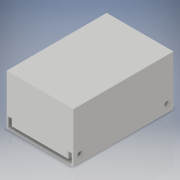
# Autodesk Inventor part: Case
Saved by Autodesk Inventor 2019 (Build 230136000, 136)
## iProperties
Created: 2019-12-10
Part Number: Case
Material: 常规
Document SubType Name: Modeling
Designer: cxcyh
Density: 1 g/cm^3
Appearance: 默认
Author: cxcyh
Autodesk Inventor part; units mm, degrees
ref_plane "YZ Plane" through (0, 0, 0) normal (1, 0, 0) x (0, 1, 0)
ref_plane "XZ Plane" through (0, 0, 0) normal (0, 1, 0) x (-1, 0, 0)
ref_plane "XY Plane" through (0, 0, 0) normal (0, 0, 1) x (1, 0, 0)
sketch "草图2" plane through (0, 0, 0) normal (0, 1, 0) x (-1, 0, 0)
  line L0 (-20, 30) -> (20, 30)
  line L1 (20, 30) -> (20, -30)
  line L2 (20, -30) -> (-20, -30)
  line L3 (-20, -30) -> (-20, 30)
  line L4 (-20, 30) -> (20, -30) construction
  line L5 (20, 30) -> (-20, -30) construction
  point P0 (0, 0)
  dimension "d15" = 40
  dimension "d16" = 60
  constraints: 12 end point, 2 midpoint, 2 parallel, 1 horizontal, 1 perpendicular
  measures "d15" distance of L1.end L2.end
  measures "d16" distance of L0.end L1.end
extrude "拉伸2" add sketch "草图2" along normal blind 30
shell "抽壳1" thickness 2 removed faces 1 at (-6.6667, 0, -10)
sketch "草图3" plane through (-20, 0, 30) normal (0, 0, 1) x (1, 0, 0)
  line L0 (40, 0) -> (0, 0) construction
  line L1 (40, 0) -> (40, 30) construction
  line L2 (0, 30) -> (40, 30) construction
  line L3 (0, 0) -> (0, 30) construction
  line L4 (0, 0) -> (0, 30) construction
  line L5 (40, 0) -> (40, 30) construction
  line L6 (40, 0) -> (0, 0) construction
  line L7 (3, 6.7398) -> (1, 6.7398)
  line L8 (1, 6.7398) -> (1, 0.7398)
  line L9 (0, 1.7398) -> (40, 1.7398) construction
  line L10 (3, 6.7398) -> (3, 2.7398)
  line L11 (40, 30) -> (0, 30) construction
  line L12 (20, 30) -> (20, 0) construction
  line L13 (38, 0) -> (2, 0) projected
  line L14 (3, 2.7398) -> (20, 2.7398)
  line L15 (1, 0.7398) -> (20, 0.7398)
  line L16 (37, 6.7398) -> (39, 6.7398)
  line L17 (39, 6.7398) -> (39, 0.7398)
  line L18 (37, 6.7398) -> (37, 2.7398)
  line L19 (37, 2.7398) -> (20, 2.7398)
  line L20 (39, 0.7398) -> (20, 0.7398)
  point P0 (20, 0)
  dimension "d29" = 2
  dimension "d44" = 5
  dimension "d45" = 2
  dimension "d46" = 6
  dimension "d47" = 40
  constraints: 24 end point, 5 point on line, 4 symmetric about line, 3 horizontal, 3 perpendicular, 2 midpoint
  measures "d29" distance from line of L7.start L8
  measures "d44" distance between parallel lines of L9 L7
  measures "d45" distance between parallel lines of L15 L14
  measures "d46" distance between parallel lines of L15 L7
  measures "d47" diameter of L1 L12
extrude "拉伸3" cut sketch "草图3" against normal blind 58
sketch "草图5" plane through (20, 0, 30) normal (1, 0, 0) x (0, 0, -1)
  line L0 (0, 6.7398) -> (58, 6.7398) construction
  line L1 (0, 0.7398) -> (58, 0.7398) construction
  line L2 (0, 6.7398) -> (2, 6.7398) construction
  line L3 (0, 2.7398) -> (2, 2.7398) construction
  line L4 (0, 2.7398) -> (58, 2.7398) construction
  line L5 (58, 6.7398) -> (2, 6.7398) construction
  line L6 (58, 6.7398) -> (58, 0.7398) construction
  line L7 (0, 0) -> (0, 30) construction
  line L8 (0, 4.7398) -> (58, 4.7398) construction
  circle A0 centre (4, 4.7398) radius 1.5
  line L9 (2, 0.7398) -> (2, 6.7398) construction
  circle A1 centre (56, 4.7398) radius 1.5
  point P0 (30, 0)
  dimension "d48" = 4
  dimension "d49" = 3
  dimension "d51" = 2
  dimension "d52" = 2
  dimension "d53" = 3
  dimension "d54" = 2
  constraints: 8 end point, 6 point on line, 3 perpendicular, 2 centre point, 1 horizontal
  measures "d48" diameter of L0 L8
  measures "d49" diameter of A0
  measures "d51" distance between parallel lines of L7 L9
  measures "d52" distance from line of A0.centre L9
  measures "d53" diameter of A1
  measures "d54" distance of L8.end A1.centre
extrude "拉伸4" cut sketch "草图5" against normal blind 2
mirror "镜像1" about plane through (0, 0, 0) normal (1, 0, 0) of "拉伸4"
sketch "草图7" plane through (-18, 28, 28) normal (0, -1, 0) x (1, 0, 0)
  line L0 (0, 0) -> (36, 0) construction
  line L1 (0, -56) -> (0, 0) construction
  line L2 (36, -56) -> (0, -56) construction
  line L3 (36, 0) -> (36, -56) construction
  line L4 (0.5, -55.5) -> (18.5, -55.5) construction
  line L5 (18.5, -55.5) -> (18.5, -10.5) construction
  line L6 (18.5, -10.5) -> (0.5, -10.5) construction
  line L7 (0.5, -10.5) -> (0.5, -55.5) construction
  circle A0 centre (1.5, -54.5) radius 0.9
  line L8 (3, -56) -> (0, -56)
  line L9 (0, -56) -> (0, -53)
  line L10 (0, -53) -> (3, -53)
  line L11 (3, -53) -> (3, -56)
  line L12 (3, -56) -> (0, -53) construction
  line L13 (0, -56) -> (3, -53) construction
  line L14 (0.5, -55.5) -> (18.5, -10.5) construction
  line L15 (0.5, -10.5) -> (18.5, -55.5) construction
  line L16 (3, -13) -> (0, -13)
  line L17 (0, -13) -> (0, -10)
  line L18 (0, -10) -> (3, -10)
  line L19 (3, -10) -> (3, -13)
  circle A1 centre (1.5, -11.5) radius 0.9
  line L20 (19, -56) -> (16, -56)
  line L21 (16, -56) -> (16, -53)
  line L22 (16, -53) -> (19, -53)
  line L23 (19, -53) -> (19, -56)
  circle A2 centre (17.5, -54.5) radius 0.9
  line L24 (19, -13) -> (16, -13)
  line L25 (16, -13) -> (16, -10)
  line L26 (16, -10) -> (19, -10)
  line L27 (19, -10) -> (19, -13)
  circle A3 centre (17.5, -11.5) radius 0.9
  point P0 (9.5, -33)
  dimension "d70" = 18
  dimension "d71" = 45
  dimension "d79" = 1.8
  dimension "d80" = 1
  dimension "d81" = 1
  dimension "d82" = 3
  dimension "d83" = 3
  dimension "d91" = 43
  dimension "d94" = 16
  dimension "d97" = 1
  dimension "d98" = 1
  constraints: 48 end point, 4 centre point, 4 parallel, 3 horizontal, 3 midpoint, 2 perpendicular, 1 vertical, 30 other
  measures "d70" distance of L6.end L5.end
  measures "d71" distance of L5.end L4.end
  measures "d79" diameter of A0
  measures "d80" distance from line of L7 A0.centre
  measures "d81" distance from line of L4 A0.centre
  measures "d82" distance of L9.end L10.end
  measures "d83" distance of L8.end L9.end
  measures "d91" distance of L8.start L16.start
  measures "d94" distance of L8.start L20.start
  measures "d97" distance from line of L5 A2.centre
  measures "d98" distance from line of L6 A3.centre
sketch "草图9" plane through (20, 0, -30) normal (0, 0, -1) x (-1, 0, 0)
  line L0 (37.5, 28) -> (19.5, 28) construction
  line L1 (32, 24.8) -> (25, 24.8)
  line L2 (25, 24.8) -> (25, 28)
  line L3 (25, 28) -> (32, 28)
  line L4 (32, 28) -> (32, 24.8)
  line L5 (32, 24.8) -> (25, 28) construction
  line L6 (25, 24.8) -> (32, 28) construction
  point P0 (20, 0)
  point P1 (28.5, 26.4)
  dimension "d99" = 18
  dimension "d100" = 7
  dimension "d101" = 3.2
  dimension "d102" = 1.6
  dimension "d103" = 9
  constraints: 12 end point, 2 midpoint, 2 parallel, 1 horizontal, 1 perpendicular
  measures "d99" distance of L0.start L0.end
  measures "d100" distance of L2.end L3.end
  measures "d101" distance of L1.end L2.end
  measures "d102" distance from line of L0 point (28.5, 26.4)
  measures "d103" horizontal distance of L0.end point (28.5, 26.4)
extrude "拉伸5" add sketch "草图7" along normal blind 3.2
extrude "拉伸6" cut sketch "草图9" against normal blind 2
sketch "草图10" plane through (20, 0, -30) normal (0, 0, -1) x (-1, 0, 0)
  line L0 (32, 28) -> (32, 24.8) construction
  line L1 (32, 24.8) -> (25, 24.8) construction
  line L2 (25, 24.8) -> (25, 28) construction
  line L3 (25, 28) -> (32, 28) construction
  line L4 (40, 0) -> (0, 0) construction
  line L5 (40, 0) -> (40, 30) construction
  line L6 (0, 30) -> (40, 30) construction
  line L7 (0, 0) -> (0, 30) construction
  line L8 (25, 28) -> (25, 24.8) construction
  line L9 (25, 24.8) -> (32, 24.8) construction
  line L10 (32, 24.8) -> (32, 28) construction
  line L11 (32, 28) -> (35, 28) construction
  line L12 (35, 28) -> (35, 24.8) construction
  line L13 (35, 24.8) -> (38, 24.8) construction
  line L14 (38, 6.7398) -> (38, 24.8) construction
  line L15 (39, 6.7398) -> (38, 6.7398) construction
  line L16 (39, 0.7398) -> (39, 6.7398) construction
  line L17 (38, 0.7398) -> (39, 0.7398) construction
  line L18 (38, 0) -> (38, 0.7398) construction
  line L19 (2, 0) -> (38, 0) construction
  line L20 (2, 0) -> (2, 0.7398) construction
  line L21 (1, 0.7398) -> (2, 0.7398) construction
  line L22 (1, 6.7398) -> (1, 0.7398) construction
  line L23 (2, 6.7398) -> (1, 6.7398) construction
  line L24 (2, 6.7398) -> (2, 28) construction
  line L25 (2, 28) -> (19, 28) construction
  line L26 (19, 28) -> (19, 24.8) construction
  line L27 (19, 24.8) -> (22, 24.8) construction
  line L28 (22, 24.8) -> (22, 28) construction
  line L29 (22, 28) -> (25, 28) construction
  circle A0 centre (10.5, 11.2398) radius 7.5
  line L30 (37, 2.7398) -> (3, 2.7398) construction
  line L31 (38, 28) -> (2, 28) construction
  line L32 (10.5, 28) -> (10.5, 0) construction
  line L33 (2, 0) -> (38, 0) construction
  line L34 (5.25, 21.5) -> (15.75, 21.5)
  line L35 (15.75, 21.5) -> (15.75, 26)
  line L36 (15.75, 26) -> (5.25, 26)
  line L37 (5.25, 26) -> (5.25, 21.5)
  line L38 (5.25, 21.5) -> (15.75, 26) construction
  line L39 (15.75, 21.5) -> (5.25, 26) construction
  line L40 (28.5, 24.8) -> (28.5, 2.7398) construction
  line L41 (26.25, 3.9898) -> (30.75, 3.9898)
  line L42 (30.75, 3.9898) -> (30.75, 5.4898)
  line L43 (30.75, 5.4898) -> (26.25, 5.4898)
  line L44 (26.25, 5.4898) -> (26.25, 3.9898)
  line L45 (26.25, 3.9898) -> (30.75, 5.4898) construction
  line L46 (30.75, 3.9898) -> (26.25, 5.4898) construction
  point P0 (20, 0)
  point P1 (10.5, 23.75)
  point P2 (28.5, 4.7398)
  dimension "d108" = 15
  dimension "d111" = 8.5
  dimension "d112" = 17
  dimension "d113" = 10.5
  dimension "d114" = 4.5
  dimension "d115" = 2
  dimension "d116" = 4.5
  dimension "d117" = 1.5
  dimension "d118" = 2
  constraints: 28 end point, 5 midpoint, 5 point on line, 4 parallel, 4 perpendicular, 2 horizontal, 1 centre point, 2 other
  measures "d108" diameter of A0
  measures "d111" distance from line of L30 A0.centre
  measures "d112" diameter of L24 L32
  measures "d113" distance of L36.end L35.end
  measures "d114" distance of L35.end L34.end
  measures "d115" distance between parallel lines of L36 L25
  measures "d116" distance of L43.end L42.end
  measures "d117" distance of L42.end L41.end
  measures "d118" distance from line of L30 point (28.5, 4.74)
extrude "拉伸7" cut sketch "草图10" against normal blind 2
equation "\"d102\" = 0.5 * d101"
equation "\"d103\" = 0.5 * d99"
